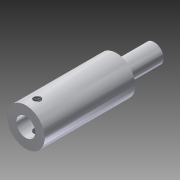
# Autodesk Inventor part: Extender
Saved by Autodesk Inventor 2015 (Build 190159000, 159)
## iProperties
Created: 2015-01-06
Part Number: Extender
Material: Aluminum 6061
Document SubType Name: Modeling
Designer: ice
Mass: 1.90852 g
Surface Area: 13.1319 cm^2
Volume: 1.90852 cm^3
Density: 2.7 g/cm^3
Appearance: Aluminum - Flat
Author: ice
Autodesk Inventor part; units mm, degrees
ref_plane "YZ Plane" through (0, 0, 0) normal (1, 0, 0) x (0, 1, 0)
ref_plane "XZ Plane" through (0, 0, 0) normal (0, 1, 0) x (-1, 0, 0)
sketch "Sketch1" plane through (0, 0, 0) normal (1, 0, 0) x (0, 1, 0)
  line L0 (0, 2.5) -> (-4, 2.5)
  line L1 (-4, 2.5) -> (-4, 5)
  line L2 (-4, 5) -> (2, 5)
  line L3 (30, 2.5) -> (20, 2.5)
  line L4 (20, 2.5) -> (20, 5)
  line L5 (20, 5) -> (2, 5)
  line L6 (30, 1) -> (0, 1)
  line L7 (0, 0) -> (31.6248, 0)
  arc A0 (30, 2.2) -> (30, 1.3) centre (30, 1.75) ccw
  line L8 (30, 1.25) -> (30, 1.3)
  line L9 (30, 2.2) -> (30, 2.25)
  line L10 (30, 1) -> (30, 1.3)
  line L11 (30, 2.2) -> (30, 2.5)
  arc A1 (0, 1.3) -> (0, 2.2) centre (0, 1.75) ccw
  line L12 (0, 1) -> (0, 1.3)
  line L13 (0, 2.2) -> (0, 2.5)
  line L14 (0, 1.25) -> (0, 1.3)
  line L15 (0, 2.2) -> (0, 2.25)
  line L16 (-4, 5) -> (0, 5)
  dimension "d0" = 2.5
  dimension "d1" = 4
  dimension "d2" = 2.5
  dimension "d6" = 10
  dimension "d7" = 2.5
  dimension "d32" = 0.9
  dimension "d33" = 0.3
  dimension "d34" = 1.75
  dimension "d35" = 0.9
  dimension "d36" = 2.5
  dimension "d37" = 1.75
  dimension "d38" = 4
  dimension "d39" = 20
  constraints: 34 end point, 9 perpendicular, 5 point on line, 4 point on circle, 4 vertical, 2 centre point, 1 horizontal
  measures "d0" distance of L7.start L0.start
  measures "d1" distance of L0.start L0.end
  measures "d2" distance of L0.end L1.end
  measures "d6" distance of L3.start L3.end
  measures "d7" distance of L3.end L4.end
  measures "d32" distance of L13.start L12.end
  measures "d33" distance of L0.start L13.start
  measures "d34" distance of L7.start A1.centre
  measures "d35" distance of L9.start L8.end
  measures "d36" distance from line of L7 L3.start
  measures "d37" distance from line of L7 A0.centre
  measures "d38" distance of L1.end L16.end
  measures "d39" distance of L4.end L16.end
revolve "Revolution1" add sketch "Sketch1" angle 360 about axis through (0, 0, 0) along (0, 1, 0)
ref_plane "Work Plane2" through (0, 0, 5) normal (0, 0, 1) x (1, 0, 0)
sketch "Sketch5" plane through (0, 0, 5) normal (0, 0, 1) x (1, 0, 0)
  line L0 (5, -4) -> (-5, -4) projected
  point P0 (0, -1)
hole "Hole1" at (0, -1, 5) direction (0, 0, -1) diameter 1.9 end through all
thread "Thread1" size "M2x0.4" class "6H" standard "ANSI Metric M Profile" full length
thread "Thread2" size "M2x0.4" class "6H" standard "ANSI Metric M Profile" full length
body "Solid1"
